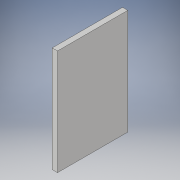
# Autodesk Inventor part: plaque
Saved by Autodesk Inventor 2017 (Build 210142000, 142)
## iProperties
Created: 2018-11-10
Part Number: plaque
Material: Generic
Document SubType Name: Modeling
Designer: Antoine Blaud
Density: 1 g/cm^3
Appearance: Default
Author: Antoine Blaud
Autodesk Inventor part; units mm, degrees
ref_plane "YZ Plane" through (0, 0, 0) normal (1, 0, 0) x (0, 1, 0)
ref_plane "XZ Plane" through (0, 0, 0) normal (0, 1, 0) x (-1, 0, 0)
ref_plane "XY Plane" through (0, 0, 0) normal (0, 0, 1) x (1, 0, 0)
sketch "Sketch1" plane through (0, 0, 0) normal (1, 0, 0) x (0, 1, 0)
  line L0 (-20, 13.335) -> (20, 13.335)
  line L1 (20, 13.335) -> (20, -13.335)
  line L2 (20, -13.335) -> (-20, -13.335)
  line L3 (-20, -13.335) -> (-20, 13.335)
  line L4 (-20, 13.335) -> (20, -13.335) construction
  line L5 (20, 13.335) -> (-20, -13.335) construction
  point P0 (0, 0)
  dimension "d2" = 40
  dimension "d3" = 26.67
  constraints: 12 end point, 2 midpoint, 2 parallel, 1 horizontal, 1 perpendicular
  measures "d2" distance of L1.end L2.end
  measures "d3" distance of L0.end L1.end
extrude "Extrusion1" add sketch "Sketch1" along normal blind 2
body "Solid1"
